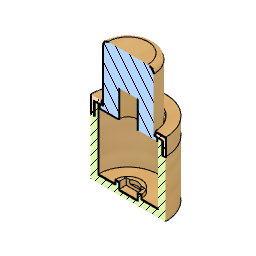
Probatio Assembly 1.0 v9 (Autodesk Fusion 360 archive; units mm, degrees)
design "Button_Hall_2.0_Parametric"
Autodesk Fusion 360 part; units mm, degrees
sketch "Sketch1" plane through (0, 0, 0) normal (0, 1, 0) x (1, 0, 0) in component "Base"
  circle A0 centre (0, 0) radius 10
  dimension "d63" = 20
  constraint coincident A0.centre origin
  measures "d63" diameter of A0
extrude "Extrude1" add sketch "Sketch1" along normal blind 2 makes body 1 in component "Base"
sketch "Sketch2" plane through (0, 2, 0) normal (0, 1, 0) x (-1, 0, 0) in component "Base"
  circle A0 centre (0, 0) radius 10
  circle A1 centre (0, 0) radius 8
  dimension "d66" = -2
extrude "Extrude2" add sketch "Sketch2" along normal blind 13 bodies 1 in component "Base"
sketch "Sketch3" plane through (0, 15, 0) normal (0, 1, 0) x (-1, 0, 0) in component "Base"
  circle A0 centre (0, 0) radius 8
  circle A1 centre (0, 0) radius 10
  circle A2 centre (0, 0) radius 9
  dimension "d69" = 1
extrude "Extrude3" add sketch "Sketch3" along normal blind 3.5 contours A2 bodies 1 in component "Base"
sketch "Sketch2 (2)" plane through (0, 15, 0) normal (0, 1, 0) x (-1, 0, 0) in component "Ring"
  circle A0 centre (0, 0) radius 9 construction
  circle A1 centre (0, 0) radius 10
  circle A2 centre (0, 0) radius 9.2
  dimension "offset_bottom" = 0.2
extrude "Extrude1'" add sketch "Sketch2 (2)" along normal blind 3.5 separate body makes body 2 in component "Ring"
sketch "Sketch3 (2)" plane through (0, 18.5, 0) normal (0, 1, 0) x (-1, 0, 0) in component "Ring"
  circle A0 centre (0, 0) radius 9.2 construction
  circle A1 centre (0, 0) radius 10
extrude "Extrude2'" add sketch "Sketch3 (2)" along normal blind 1 bodies 2 in component "Ring"
sketch "Sketch4" plane through (0, 19.5, 0) normal (0, 1, 0) x (-1, 0, 0) in component "Ring"
  circle A0 centre (0, 0) radius 10
  circle A1 centre (0, 0) radius 9
  circle A2 centre (0, 0) radius 7.2
  dimension "d77" = 18
  dimension "diameter_apperture" = 14.4
  constraint coincident A0.centre A1.centre
  constraint concentric A1 A2
  measures "d77" diameter of A1
  measures "diameter_apperture" diameter of A2
extrude "Extrude3'" cut sketch "Sketch4" against normal blind 1 contours A2 bodies 2 in component "Ring"
sketch "Sketch1 (2)" plane through (0, 18.5, 0) normal (0, -1, 0) x (1, 0, 0) in component "Top"
  circle A0 centre (0, 0) radius 7.2 construction
  circle A1 centre (0, 0) radius 9.2 construction
  circle A2 centre (0, 0) radius 7.7
  dimension "diameter_bottom_disc" = 15.4
  constraint concentric A0 A2
  measures "diameter_bottom_disc" diameter of A2
extrude "Extrude1''" add sketch "Sketch1 (2)" along normal blind 1 separate body makes body 3 in component "Top"
ref_plane "WorkPlane2" through (0, 17.1186, 0) normal (0, 0, 1) x (-1, 0, 0)
sketch "Sketch2 (3)" plane through (0, 18.5, 0) normal (0, 1, 0) x (-1, 0, 0) in component "Top"
  circle A0 centre (0, 0) radius 7.7
  circle A1 centre (0, 0) radius 6.8
  dimension "diameter_tower" = 13.6
  constraint concentric A0 A1
  measures "diameter_tower" diameter of A1
extrude "Extrude2''" add sketch "Sketch2 (3)" along normal blind 15.5 contours A1 bodies 3 in component "Top"
sketch "Sketch3 (3)" plane through (0, 17.5, 0) normal (0, -1, 0) x (1, 0, 0) in component "Top"
  circle A0 centre (0, 0) radius 7.7
  circle A1 centre (0, 0) radius 2.5
  dimension "d90" = 5
  constraint coincident A0.centre A1.centre
  measures "d90" diameter of A1
extrude "Extrude3''" cut sketch "Sketch3 (3)" against normal blind 7.2 contours A1 bodies 3 in component "Top"
sketch "Sketch4 (2)" plane through (0, 2, 0) normal (0, 1, 0) x (-1, 0, 0) in component "Base"
  circle A0 centre (0, 0) radius 8
  circle A1 centre (0, 0) radius 2.5
  circle A2 centre (0, 0) radius 3.5
  dimension "d98" = 5
  dimension "d99" = 1
  constraint concentric A0 A1
  measures "d98" diameter of A1
extrude "Extrude4" add sketch "Sketch4 (2)" along normal blind 1 contours A2 bodies 1 in component "Base"
ref_plane "WorkPlane1" through (0, 2.8235, -3.5) normal (0, 0, -1) x (1, 0, 0) in component "Base"
ref_plane "WorkPlane2" through (0, 2.5, 3.5) normal (0, 0, 1) x (1, 0, 0) in component "Base"
ref_plane "WorkPlane3" through (0, 2.8235, 0) normal (0, 0, -1) x (1, 0, 0) in component "Base"
sketch "Sketch6" plane through (0, 2.8235, 0) normal (0, 0, -1) x (1, 0, 0) in component "Base"
  line L0 (-3.5, -0.1765) -> (3.5, -0.1765)
  line L1 (-10, 2.8235) -> (10, 2.8235)
  line L2 (3.5, 0.8235) -> (-3.5, 0.8235) construction
  line L3 (-3.5, -0.1765) -> (-3.5, 0.8235) construction
  line L4 (3.5, -0.1765) -> (3.5, 0.8235) construction
  line L5 (-3.5, -0.1765) -> (-2.5, -0.1765) construction
  line L6 (-2.5, -0.1765) -> (-2.5, 0.8235) construction
  line L7 (-2.5, 0.8235) -> (-3.5, 0.8235) construction
  line L8 (-3.5, 0.8235) -> (-3.5, -0.1765) construction
  line L9 (3.5, -0.1765) -> (2.5, -0.1765) construction
  line L10 (2.5, -0.1765) -> (2.5, 0.8235) construction
  line L11 (2.5, 0.8235) -> (3.5, 0.8235) construction
  line L12 (3.5, 0.8235) -> (3.5, -0.1765) construction
  line L13 (-2.5, -0.1765) -> (2.5, -0.1765)
  line L14 (2.5, -0.1765) -> (2.5, 1.6235)
  line L15 (2.5, 1.6235) -> (-2.5, 1.6235)
  line L16 (-2.5, 1.6235) -> (-2.5, -0.1765)
  dimension "d104" = 1
  dimension "d105" = 1
  dimension "d106" = 1
  dimension "d107" = 1
  dimension "d108" = 1.8
  constraint coincident L0.start L3.start
  constraint coincident L2.end L3.end
  constraint coincident L0.end L4.start
  constraint coincident L2.start L4.end
  constraint horizontal L5
  constraint vertical L6
  constraint horizontal L7
  constraint vertical L8
  constraint horizontal L9
  constraint vertical L10
  constraint horizontal L11
  constraint vertical L12
  constraint perpendicular L13 L14
  constraint parallel L13 L15
  constraint parallel L14 L16
  measures "d104" distance of L0.start L2.end
  measures "d105" distance of L0.start L5.end
  measures "d106" distance of L0.end L9.end
  measures "d107" distance of L0.end L2.start
  measures "d108" distance of L5.end L15.end
extrude "Extrude5" cut sketch "Sketch6" along normal blind 2 bodies 1 in component "Base"
extrude "Extrude6" cut sketch "Sketch6" against normal through all bodies 1 in component "Base"
ref_plane "WorkPlane4" through (0, 2.8235, 2) normal (0, 0, -1) x (1, 0, 0) in component "Base"
sketch "Sketch7" plane through (0, 2.8235, 2) normal (0, 0, -1) x (1, 0, 0) in component "Base"
  line L0 (2.5, -0.1765) -> (2.5, 1.6235)
  line L1 (-2.5, -0.1765) -> (2.5, -0.1765)
  line L2 (2.5, 1.6235) -> (-2.5, 1.6235)
  line L3 (-2.5, 1.6235) -> (-2.5, -0.1765)
extrude "Extrude7" cut sketch "Sketch7" against normal through all draft 5 bodies 1 in component "Base"
fillet "Fillet1" radius 1.5 1 edges at (6.3398, 34, -2.459) on bodies 3 in component "Top"
component "Base" placed x (1, 0, 0) y (0, 1, 0) z (0, 0, 1) at (0, 0, 0)
component "Ring" placed x (1, 0, 0) y (0, 1, 0) z (0, 0, 1) at (0, 0, 0)
component "Top" placed x (1, 0, 0) y (0, 1, 0) z (0, 0, 1) at (0, 0, 0)
equation "base_diameter = 20 mm"
equation "tolerance = 0.2 mm"
equation "wall_thickness = 1 mm"
equation "base_total_height = 18.5 mm"
equation "base_ring_height = 3.5 mm"
equation "base_bottom_thickness = 2 mm"
equation "d63 = base_diameter"
equation "d64 = base_bottom_thickness"
equation "d66 = -2 * wall_thickness"
equation "d67 = base_total_height - base_bottom_thickness - base_ring_height"
equation "d69 = wall_thickness"
equation "d70 = base_ring_height"
equation "offset_bottom = tolerance"
equation "d73 = base_ring_height"
equation "d75 = wall_thickness"
equation "d77 = base_diameter - 2 * wall_thickness"
equation "diameter_apperture = base_diameter - 6 * wall_thickness + 2 * tolerance"
equation "d79 = -wall_thickness"
equation "diameter_bottom_disc = base_diameter - 4 * wall_thickness - 3 * tolerance"
equation "d83 = wall_thickness"
equation "diameter_tower = base_diameter - 6 * wall_thickness - 2 * tolerance"
equation "top_safety_margin = 1 mm" comment "To avoid the top to get stuck inside base"
equation "d88 = base_total_height - 2 * wall_thickness - base_bottom_thickness + top_safety_margin"
equation "d90 = magnet_diameter"
equation "magnet_diameter = 5 mm"
equation "magnet_height = 2.4 mm"
equation "magnet_quantity = 3"
equation "d95 = -magnet_height * magnet_quantity"
equation "spring_diameter = 5 mm"
equation "d98 = spring_diameter"
equation "d99 = wall_thickness"
equation "d100 = wall_thickness"
equation "d104 = wall_thickness"
equation "d105 = wall_thickness"
equation "d106 = wall_thickness"
equation "d107 = wall_thickness"

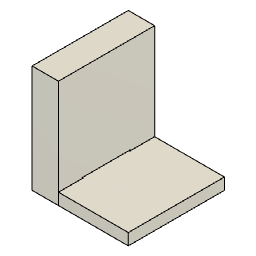
design "Side-ways support"
Autodesk Fusion 360 part; units mm, degrees
sketch "Sketch1" plane through (0, 0, 0) normal (0, 1, 0) x (1, 0, 0)
  line L0 (25, -25) -> (-25, -25)
  line L1 (-25, -25) -> (-25, 25)
  line L2 (-25, 25) -> (25, 25)
  line L3 (25, 25) -> (25, -25)
  line L4 (25, -25) -> (-25, 25) construction
  line L5 (-25, -25) -> (25, 25) construction
  dimension "d1" = 50
  dimension "d2" = 50
  constraint perpendicular L0 L1
  constraint parallel L0 L2
  constraint parallel L1 L3
  constraint horizontal L0
  constraint coincident L4 origin
  constraint coincident L5 origin
  measures "d1" distance of L1.end L2.end
  measures "d2" distance of L0.end L1.end
extrude "Extrude1" add sketch "Sketch1" along normal blind 6 makes body 1
sketch "Sketch2" plane through (0, 6, 0) normal (0, 1, 0) x (-1, 0, 0)
  line L0 (-25, -25) -> (25, -25)
  line L1 (25, -25) -> (25, 25)
  line L2 (25, 25) -> (-25, 25)
  line L3 (-25, 25) -> (-25, -25)
  line L4 (25, -25) -> (11.3, -25)
  line L5 (11.3, -25) -> (11.3, 25)
  line L6 (11.3, 25) -> (25, 25)
  line L7 (25, 25) -> (25, -25)
  dimension "d5" = 50
  dimension "d6" = 13.7
  constraint horizontal L4
  constraint vertical L5
  constraint horizontal L6
  constraint vertical L7
  constraint coincident L0.end L1.start
  measures "d5" distance of L0.end L1.end
  measures "d6" distance of L0.end L4.end
extrude "Extrude2" add sketch "Sketch2" along normal blind 50 contours L0 L1 L2 L4 L5 L6 L7 bodies 1
sketch "Sketch3" plane through (-25, 0, 0) normal (-1, 0, 0) x (0, 0, 1)
  line L0 (-25, 0) -> (25, 0)
  line L1 (25, 0) -> (25, 56)
  line L2 (25, 56) -> (-25, 56)
  line L3 (-25, 56) -> (-25, 0)
  line L4 (-23, 2) -> (23, 2)
  line L5 (23, 2) -> (23, 54)
  line L6 (23, 54) -> (-23, 54)
  line L7 (-23, 54) -> (-23, 2)
  dimension "d9" = -2
extrude "Extrude3" cut sketch "Sketch3" against normal blind 12 contours L4 L5 L6 L7 bodies 1
sketch "Sketch4" plane through (-13, 0, 0) normal (-1, 0, 0) x (0, 0, 1)
  line L0 (-23, 54) -> (-23, 2)
  line L1 (-23, 2) -> (23, 2)
  line L2 (23, 2) -> (23, 54)
  line L3 (23, 54) -> (-23, 54)
  line L4 (23, 2) -> (-23, 2) construction
  line L5 (-23, 2) -> (-23, 5) construction
  line L6 (-23, 5) -> (23, 5) construction
  line L7 (23, 5) -> (23, 2) construction
  line L8 (-23, 54) -> (23, 54) construction
  line L9 (23, 54) -> (23, 8) construction
  line L10 (23, 8) -> (-23, 8) construction
  line L11 (-23, 8) -> (-23, 54) construction
  line L12 (-23, 54) -> (23, 8) construction
  line L13 (23, 54) -> (-23, 8) construction
  line L14 (11, 20) -> (-11, 20) construction
  line L15 (-11, 20) -> (-11, 42) construction
  line L16 (-11, 42) -> (11, 42) construction
  line L17 (11, 42) -> (11, 20) construction
  line L18 (11, 20) -> (-11, 42) construction
  line L19 (-11, 20) -> (11, 42) construction
  circle A0 centre (-11, 42) radius 6.25
  circle A1 centre (11, 42) radius 6.25
  circle A2 centre (-11, 20) radius 6.25
  circle A3 centre (11, 20) radius 6.25
  point P0 (0, 31)
  dimension "d14" = 46
  dimension "d15" = 3
  dimension "d16" = 46
  dimension "d17" = 46
  dimension "d18" = 22
  dimension "d19" = 22
  dimension "d20" = 12.5
  dimension "d23" = 22
  dimension "d24" = -22
  constraint horizontal L4
  constraint vertical L5
  constraint horizontal L6
  constraint vertical L7
  constraint coincident L1.end L2.start
  constraint horizontal L8
  constraint vertical L9
  constraint horizontal L10
  constraint vertical L11
  constraint coincident L0.start L3.end
  constraint coincident L2.end L3.start
  constraint perpendicular L14 L15
  constraint parallel L14 L16
  constraint parallel L15 L17
  constraint horizontal L14
  constraint coincident L18 P0
  constraint coincident L19 P0
  constraint midpoint L12 P0
  constraint coincident L15.end L16.start
  measures "d14" distance of L1.end L0.end
  measures "d15" distance of L1.end L6.end
  measures "d16" distance of L0.start L2.end
  measures "d17" distance of L0.start L10.end
  measures "d18" distance of L15.end L16.end
  measures "d19" distance of L14.end L15.end
  measures "d20" diameter of A0
extrude "Extrude4" cut sketch "Sketch4" against normal blind 1 contours A0 | A1 | A2 | A3 bodies 1
split "Split1" by plane through (-11.3, 6, -25) normal (1, 0, 0) bodies 1 makes body 2 at (12.9, 0, 8.3333)
sketch "Sketch5" plane through (-11.3, 0, 0) normal (-1, 0, 0) x (0, 0, 1)
  line L0 (25, 6) -> (-25, 6)
  line L1 (-25, 6) -> (-25, 0)
  line L2 (-25, 0) -> (25, 0)
  line L3 (25, 0) -> (25, 6)
  line L4 (-25, 6) -> (25, 6)
  line L5 (25, 6) -> (25, 3)
  line L6 (25, 3) -> (-25, 3)
  line L7 (-25, 3) -> (-25, 6)
  line L8 (0, 6) -> (0, 3) construction
  line L9 (12.5, 3.4) -> (-12.5, 3.4) construction
  line L10 (-12.5, 3.4) -> (-12.5, 6.4) construction
  line L11 (-12.5, 6.4) -> (12.5, 6.4) construction
  line L12 (12.5, 6.4) -> (12.5, 3.4) construction
  line L13 (12.5, 3.4) -> (-12.5, 6.4) construction
  line L14 (-12.5, 3.4) -> (12.5, 6.4) construction
  line L15 (-12.1, 3.8) -> (-12.1, 6)
  line L16 (-12.1, 6) -> (12.1, 6)
  line L17 (12.1, 6) -> (12.1, 3.8)
  line L18 (12.1, 3.8) -> (-12.1, 3.8)
  point P0 (0, 4.5)
  dimension "d27" = 25
  dimension "d28" = 3
  dimension "d29" = 0.4
  constraint horizontal L4
  constraint vertical L5
  constraint horizontal L6
  constraint vertical L7
  constraint midpoint L3 L5.end
  constraint coincident L0.end L1.start
  constraint midpoint L0 L8.start
  constraint midpoint L6 L8.end
  constraint perpendicular L9 L10
  constraint parallel L9 L11
  constraint parallel L10 L12
  constraint horizontal L9
  constraint midpoint L8 P0
  measures "d27" distance of L10.end L11.end
  measures "d28" distance of L9.end L10.end
extrude "Extrude5" add sketch "Sketch5" along normal blind 14 contours L0 L4 L15 L16 L17 L18 bodies 2
sketch "Sketch6" plane through (-13, 0, 0) normal (-1, 0, 0) x (0, 0, 1)
  circle A0 centre (11, 42) radius 6.25
  circle A1 centre (-11, 20) radius 6.25
  circle A2 centre (-11, 42) radius 6.25
  circle A3 centre (11, 20) radius 6.25
  line L0 (-23, 54) -> (-23, 2)
  line L1 (-23, 2) -> (23, 2)
  line L2 (23, 2) -> (23, 54)
  line L3 (23, 54) -> (-23, 54)
  line L4 (12.1, 3.8) -> (12.1, 6) construction
  line L5 (12.1, 6) -> (-12.1, 6) construction
  line L6 (-12.1, 6) -> (-12.1, 3.8) construction
  line L7 (-12.1, 3.8) -> (12.1, 3.8) construction
  line L8 (12.5, 6.4) -> (-12.5, 6.4)
  line L9 (-12.5, 6.4) -> (-12.5, 3.4)
  line L10 (-12.5, 3.4) -> (12.5, 3.4)
  line L11 (12.5, 3.4) -> (12.5, 6.4)
  line L12 (-12.5, 6.4) -> (12.5, 3.4) construction
  line L13 (12.5, 6.4) -> (-12.5, 3.4) construction
  line L14 (14, 2.4) -> (-14, 2.4)
  line L15 (-14, 2.4) -> (-14, 7.4)
  line L16 (-14, 7.4) -> (14, 7.4)
  line L17 (14, 7.4) -> (14, 2.4)
  line L18 (14, 2.4) -> (-14, 7.4) construction
  line L19 (-14, 2.4) -> (14, 7.4) construction
  point P0 (0, 4.9)
  dimension "d32" = 0.4
  dimension "d33" = 28
  constraint perpendicular L14 L15
  constraint parallel L14 L16
  constraint parallel L15 L17
  constraint horizontal L14
  constraint coincident L18 P0
  constraint coincident L19 P0
  constraint midpoint L12 P0
  measures "d33" distance of L15.end L16.end
extrude "Extrude6" add sketch "Sketch6" along normal blind 12 contours L14 L15 L16 L17 bodies 1
extrude "Extrude7" cut 1 faces at (-13, 5.4, -4.1667) along direction (1, 0, 0) through all on bodies 1 bodies 1
extrude "Extrude8" add 1 faces at (-21, 2.4, 4.6667) along direction (0, -1, 0) blind 1 on bodies 1 bodies 1
equation "d6 = 14 mm - 0.3 mm"
